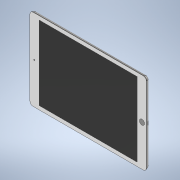
# Autodesk Inventor part: iPadModelA2197
Saved by Autodesk Inventor 2021.1 (Build 251245010, 245A)
## iProperties
Created: 2020-11-06
Part Number: iPadModelA2197
Material: 一般
Document SubType Name: Modeling
Designer: gisen
Density: 1 g/cm^3
Appearance: 滑らか - 黒
Author: gisen
Autodesk Inventor part; units mm, degrees
ref_plane "YZ Plane" through (0, 0, 0) normal (1, 0, 0) x (0, 1, 0)
ref_plane "XZ Plane" through (0, 0, 0) normal (0, 1, 0) x (-1, 0, 0)
ref_plane "XY Plane" through (0, 0, 0) normal (0, 0, 1) x (1, 0, 0)
sketch "スケッチ1" plane through (0, 0, 0) normal (0, 0, 1) x (1, 0, 0)
  line L0 (-134.0722, 55.6245) -> (115.9278, 55.6245)
  line L1 (115.9278, 55.6245) -> (115.9278, -119.3755)
  line L2 (115.9278, -119.3755) -> (-134.0722, -119.3755)
  line L3 (-134.0722, -119.3755) -> (-134.0722, 55.6245)
  point P0 (0, 0)
  dimension "d0" = 250
  dimension "d1" = 175
  constraints: 8 end point, 2 parallel, 1 horizontal, 1 perpendicular
  measures "d0" distance of L0.start L0.end
  measures "d1" distance of L0.end L1.end
extrude "押し出し1" add sketch "スケッチ1" along normal blind 8
fillet "フィレット1" radius 7 4 edges at (115.9278, 55.6245, 4) (-134.0722, 55.6245, 4) (-134.0722, -119.3755, 4) (115.9278, -119.3755, 4)
fillet "フィレット2" radius 7 8 edges at (-134.0722, -31.8755, 0) (-132.0219, -117.3252, 0) (-9.0722, -119.3755, 0) (113.8775, -117.3252, 0) (115.9278, -31.8755, 0) (113.8775, 53.5743, 0) (-9.0722, 55.6245, 0) (-132.0219, 53.5743, 0)
sketch "スケッチ2" plane through (0, 0, 8) normal (0, 0, 1) x (1, 0, 0)
  line L0 (-114.0722, 47.6245) -> (95.9278, 47.6245)
  line L1 (95.9278, 47.6245) -> (95.9278, -111.3755)
  line L2 (95.9278, -111.3755) -> (-114.0722, -111.3755)
  line L3 (-114.0722, -111.3755) -> (-114.0722, 47.6245)
  line L4 (-134.0722, 48.6245) -> (-134.0722, -112.3755) projected
  line L5 (115.9278, -112.3755) -> (115.9278, 48.6245) projected
  line L6 (108.9278, 55.6245) -> (-127.0722, 55.6245) projected
  line L7 (-127.0722, -119.3755) -> (108.9278, -119.3755) projected
  dimension "d6" = 20
  dimension "d7" = 20
  dimension "d8" = 8
  dimension "d9" = 8
  constraints: 8 end point, 2 parallel, 1 horizontal, 1 perpendicular
  measures "d6" distance between parallel lines of L4 L3
  measures "d7" distance between parallel lines of L5 L1
  measures "d8" distance between parallel lines of L6 L0
  measures "d9" distance between parallel lines of L7 L2
extrude "押し出し2" cut sketch "スケッチ2" against normal blind 0.001
sketch "スケッチ3" plane through (0, 0, 8) normal (0, 0, 1) x (1, 0, 0)
  line L0 (-127.0722, -119.3755) -> (108.9278, -119.3755) projected
  line L1 (108.9278, 55.6245) -> (-127.0722, 55.6245) projected
  circle A0 centre (106.4278, -31.8755) radius 5.5
  line L2 (115.9278, -112.3755) -> (115.9278, 48.6245) projected
  point P0 (0, 0)
  dimension "d12" = 11
  dimension "d13" = 87.5
  dimension "d14" = 9.5
  constraints: 1 centre point
  measures "d12" diameter of A0
  measures "d13" distance from line of L1 A0.centre
  measures "d14" distance from line of L2 A0.centre
extrude "押し出し3" add sketch "スケッチ3" along normal blind 0.001
sketch "スケッチ4" plane through (115.9278, -112.3755, 8) normal (1, 0, 0) x (0, 0, -1)
  line L0 (8, 0) -> (8, 161) projected
  line L1 (0, 0) -> (0, 161) projected
  line L2 (5.39, 76.72) -> (3.82, 76.72)
  line L3 (3.82, 76.72) -> (3.82, 84.28)
  line L4 (3.82, 84.28) -> (5.39, 84.28)
  line L5 (5.39, 84.28) -> (5.39, 76.72)
  point P0 (8, 112.3755)
  dimension "d17" = 1.57
  dimension "d18" = 7.56
  dimension "d19" = 3.82
  dimension "d20" = 76.72
  constraints: 8 end point, 2 parallel, 1 horizontal, 1 perpendicular
  measures "d17" distance of L2.start L2.end
  measures "d18" distance of L4.end L2.start
  measures "d19" distance between parallel lines of L3 L1
  measures "d20" distance from line of L1.end L4
extrude "押し出し4" cut sketch "スケッチ4" against normal blind 6.76
fillet "フィレット3" radius 0.5 4 edges at (112.2512, -28.0955, 4.18) (111.774, -28.0955, 2.61) (112.2512, -35.6555, 4.18) (111.774, -35.6555, 2.61)
sketch "スケッチ5" plane through (0, 0, 8) normal (0, 0, 1) x (1, 0, 0)
  circle A0 centre (-124.7722, -31.8755) radius 1.25
  line L0 (-134.0722, 48.6245) -> (-134.0722, -112.3755) projected
  line L1 (108.9278, 55.6245) -> (-127.0722, 55.6245) projected
  point P0 (0, 0)
  dimension "d24" = 2.5
  dimension "d25" = 9.3
  dimension "d26" = 87.5
  constraints: 1 centre point
  measures "d24" diameter of A0
  measures "d25" distance from line of L0 A0.centre
  measures "d26" distance from line of L1 A0.centre
extrude "押し出し5" cut sketch "スケッチ5" against normal blind 0.01
